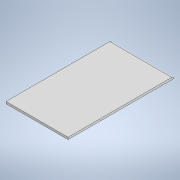
# Autodesk Inventor part: CaseCover
Saved by Autodesk Inventor 2021 (Build 250183000, 183)
## iProperties
Created: 2021-01-18
Part Number: CaseCover
Material: Generic
Document SubType Name: Modeling
Designer: Jayan
Density: 1 g/cm^3
Appearance: Default
Author: Jayan
Autodesk Inventor part; units mm, degrees
ref_plane "YZ Plane" through (0, 0, 0) normal (1, 0, 0) x (0, 1, 0)
ref_plane "XZ Plane" through (0, 0, 0) normal (0, 1, 0) x (-1, 0, 0)
ref_plane "XY Plane" through (0, 0, 0) normal (0, 0, 1) x (1, 0, 0)
sketch "Sketch1" plane through (0, 0, 0) normal (0, 1, 0) x (-1, 0, 0)
  line L0 (0, 0) -> (73.66, 0)
  line L1 (73.66, 0) -> (73.66, -125.73)
  line L2 (73.66, -125.73) -> (0, -125.73)
  line L3 (0, -125.73) -> (0, 0)
  dimension "d0" = 73.66
  dimension "d1" = 125.73
  constraints: 8 end point, 2 parallel, 1 horizontal, 1 perpendicular
  measures "d0" distance of L1.end L2.end
  measures "d1" distance of L0.end L1.end
extrude "Extrusion1" add sketch "Sketch1" along normal blind 2.54
fillet "Fillet2" radius 2.54 1 edges at (-36.83, 2.54, -125.73)
body "Solid1"
